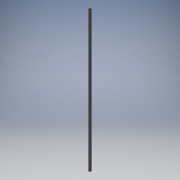
# Autodesk Inventor part: trin-rør
Saved by Autodesk Inventor 2018 (Build 220112000, 112)
## iProperties
Created: 2019-11-05
Part Number: trin-rør
Material: Steel
Document SubType Name: Modeling
Designer: loppen
Density: 7.85 g/cm^3
Appearance: Light Gray
Mass: 4534.72 g
Surface Area: 3616.58 cm^2
Volume: 577.671 cm^3
Author: loppen
Autodesk Inventor part; units mm, degrees
ref_plane "YZ Plane" through (0, 0, 0) normal (1, 0, 0) x (0, 1, 0)
ref_plane "XZ Plane" through (0, 0, 0) normal (0, 1, 0) x (-1, 0, 0)
ref_plane "XY Plane" through (0, 0, 0) normal (0, 0, 1) x (1, 0, 0)
sketch "Sketch1" plane through (0, 0, 0) normal (0, 0, 1) x (1, 0, 0)
  circle A0 centre (0, 0) radius 13.65
  circle A1 centre (0, 0) radius 16.85
  dimension "d0" = 3.2
  dimension "d1" = 33.7
  dimension "d2" = 27.3
  constraints: 2 centre point, 2 coincident
  measures "d0" radial gap between concentric circles of A1 A0
  measures "d1" diameter of A1
  measures "d2" diameter of A0
extrude "Extrusion1" add sketch "Sketch1" along normal blind 1884
equation "\"d3\" = trinbredde"
equation "\"pladetykkelse\" = 3"
equation "\"trappevinkel\" = 34.3deg"
equation "\"trappestifter_dia\" = 25"
equation "\"trappestifter_huldia\" = 25.8"
equation "\"trappestifter_skraa_huldia\" = 26.6"
equation "\"trappestifter_laengde\" = 228"
equation "\"perforeringsbredde\" = 6"
equation "\"perforeringshullaengde\" = 62.8"
equation "\"perforeringshullaengde_top\" = 61"
equation "\"perforeringshullaengde_bund\" = 61.6"
equation "\"perforeringsoffset\" = 8"
equation "\"perforeringsoffset_top\" = 8"
equation "\"perforeringsoffset_bund\" = 8"
equation "\"laskehul_dia\" = 13"
equation "\"balusterhul_udvidelse\" = 1"
equation "\"trinbredde\" = 1884"
body "Solid1"
